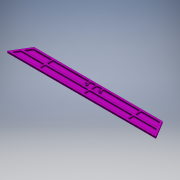
# Autodesk Inventor part: アーム　ハシゴ
Saved by Autodesk Inventor 2016 (Build 200138000, 138)
## iProperties
Created: 2016-03-06
Part Number: アーム　ハシゴ
Material: GFRP
Document SubType Name: Modeling
Designer: Takumi
Density: 1.75 g/cm^3
Appearance: 滑らか - 紫
Mass: 17.764 g
Surface Area: 193.734 cm^2
Volume: 10.1509 cm^3
Author: Takumi
Autodesk Inventor part; units mm, degrees
ref_plane "YZ Plane" through (0, 0, 0) normal (1, 0, 0) x (0, 1, 0)
ref_plane "XZ Plane" through (0, 0, 0) normal (0, 1, 0) x (-1, 0, 0)
ref_plane "XY Plane" through (0, 0, 0) normal (0, 0, 1) x (1, 0, 0)
sketch "スケッチ1" plane through (0, 0, 0) normal (0, 0, 1) x (1, 0, 0)
  line L0 (0, 0) -> (0, -14.5)
  line L1 (29.2409, -29) -> (295.7591, -29)
  line L2 (325, -16) -> (325, 0)
  line L3 (277.6805, 0.8) -> (47.3195, 0.8)
  line L4 (0, -14.5) -> (325, -14.5) construction
  arc A0 (325, -16) -> (325, -13) centre (325, -14.5) ccw
  line L5 (162.5, 0.8) -> (162.5, -29) construction
  arc A1 (161.5, -29) -> (162.5, -30) centre (162.5, -29) ccw
  line L6 (83.25, 0.8) -> (83.25, -29) construction
  arc A2 (82.25, -29) -> (83.25, -30) centre (83.25, -29) ccw
  line L7 (241.75, 0.8) -> (241.75, -29) construction
  arc A3 (240.75, -29) -> (241.75, -30) centre (241.75, -29) ccw
  line L8 (3, -3) -> (3, -13)
  line L9 (34.5698, -26) -> (82.25, -26)
  line L10 (82.25, -2.2) -> (82.25, -13)
  line L11 (82.25, -16) -> (82.25, -26)
  line L12 (84.25, -26) -> (84.25, -16)
  line L13 (84.25, -13) -> (84.25, -2.2)
  line L14 (161.5, -2.2) -> (161.5, -13)
  line L15 (161.5, -16) -> (161.5, -26)
  line L16 (163.5, -26) -> (163.5, -16)
  line L17 (163.5, -13) -> (163.5, -2.2)
  line L18 (84.25, -16) -> (161.5, -16)
  line L19 (275.9916, -2.2) -> (242.75, -2.2)
  line L20 (240.75, -2.2) -> (240.75, -13)
  line L21 (240.75, -16) -> (240.75, -26)
  line L22 (163.5, -16) -> (240.75, -16)
  line L23 (242.75, -26) -> (242.75, -16)
  line L24 (242.75, -13) -> (242.75, -2.2)
  line L25 (84.25, -26) -> (240.75, -26)
  line L26 (242.75, -26) -> (290.4302, -26)
  line L27 (322, -13) -> (322, -3)
  line L28 (150.5, 0.8) -> (150.5, -13) construction
  arc A4 (149.5, -14.5) -> (151.5, -14.5) centre (150.5, -14.5) ccw
  line L29 (174.5, -14.5) -> (174.5, 0.8) construction
  arc A5 (173.5, -14.5) -> (175.5, -14.5) centre (174.5, -14.5) ccw
  line L30 (149.5, -2.2) -> (149.5, -5.9046)
  line L31 (149.5, -11.5614) -> (149.5, -13)
  line L32 (151.5, -13) -> (151.5, -11.5614)
  line L33 (151.5, -5.9046) -> (151.5, -2.2)
  arc A6 (151.5, -11.5614) -> (151.5, -5.9046) centre (150.5, -8.733) ccw
  arc A7 (149.5, -5.9046) -> (149.5, -11.5614) centre (150.5, -8.733) ccw
  line L34 (149.5, -2.2) -> (84.25, -2.2)
  arc A8 (173.5, -5.9046) -> (173.5, -11.5614) centre (174.5, -8.733) ccw
  arc A9 (175.5, -11.5614) -> (175.5, -5.9046) centre (174.5, -8.733) ccw
  line L35 (175.5, -13) -> (175.5, -11.5614)
  line L36 (175.5, -5.9046) -> (175.5, -2.2)
  line L37 (173.5, -2.2) -> (173.5, -5.9046)
  line L38 (173.5, -11.5614) -> (173.5, -13)
  line L39 (161.5, -13) -> (151.5, -13)
  line L40 (149.5, -13) -> (84.25, -13)
  line L41 (240.75, -13) -> (175.5, -13)
  line L42 (173.5, -13) -> (163.5, -13)
  line L43 (240.75, -2.2) -> (175.5, -2.2)
  line L44 (173.5, -2.2) -> (163.5, -2.2)
  line L45 (161.5, -2.2) -> (151.5, -2.2)
  line L46 (234, 121) -> (91, 121)
  line L47 (18.0787, 0.8) -> (0, -29)
  line L48 (306.9213, 0.8) -> (325, -29)
  line L49 (162.5, 0.8) -> (162.5, 121)
  line L50 (92.6889, 118) -> (232.3111, 118)
  line L51 (40.6364, -16) -> (82.25, -16)
  line L52 (82.25, -13) -> (42.4564, -13)
  line L53 (82.25, -2.2) -> (49.0084, -2.2)
  line L54 (82.25, 100.793) -> (92.6889, 118)
  line L55 (5.3289, -26) -> (11.3956, -16)
  line L56 (13.2156, -13) -> (19.7676, -2.2)
  line L57 (282.5436, -13) -> (242.75, -13)
  line L58 (305.2324, -2.2) -> (311.7844, -13)
  line L59 (313.6044, -16) -> (319.6711, -26)
  line L60 (242.75, -16) -> (284.3636, -16)
  line L61 (342.763, -39) -> (312.551, 10.8)
  line L62 (12.449, 10.8) -> (-17.763, -39)
  line L63 (47.3195, 0.8) -> (29.2409, -29)
  line L64 (295.7591, -29) -> (277.6805, 0.8)
  line L65 (49.0084, -2.2) -> (42.4564, -13)
  line L66 (40.6364, -16) -> (34.5698, -26)
  line L67 (290.4302, -26) -> (284.3636, -16)
  line L68 (282.5436, -13) -> (275.9916, -2.2)
  point P0 (162.5, -14.5)
  point P1 (162.5, -14.1)
  point P2 (83.25, -14.1)
  point P3 (241.75, -14.1)
  point P4 (3, -24.0549)
  point P5 (322, -24.0549)
  point P6 (150.5, -7.25)
  point P7 (174.5, -6.85)
  dimension "d0" = 29
  dimension "d1" = 325
  dimension "d3" = 3
  dimension "d4" = 2
  dimension "d5" = 2
  dimension "d6" = 2
  dimension "d32" = 3
  dimension "d33" = 3
  dimension "d35" = 3
  dimension "d36" = 3
  dimension "d37" = 2
  dimension "d43" = 143
  dimension "d44" = 150
  dimension "d48" = 3
  dimension "d49" = 3
  dimension "d50" = 3
  dimension "d51" = 3
  dimension "d52" = 3
  dimension "d53" = 10
  dimension "d54" = 35
  dimension "d55" = 35
  constraints: 149 end point, 50 parallel, 30 tangent, 20 point on circle, 18 perpendicular, 18 point on line, 10 centre point, 8 midpoint, 2 coincident, 2 horizontal, 2 vertical, 1 other
  measures "d0" distance of L0.start L47.end
  measures "d1" distance of L47.end L48.end
  measures "d3" diameter of A0
  measures "d4" diameter of A1
  measures "d5" diameter of A2
  measures "d6" diameter of A3
  measures "d32" distance between parallel lines of L1 L9
  measures "d33" distance between parallel lines of L1 L25
  measures "d35" distance between parallel lines of L3 L19
  measures "d36" distance between parallel lines of L1 L26
  measures "d37" diameter of A4
  measures "d43" distance of L46.start L46.end
  measures "d44" distance between parallel lines of L1 L46
  measures "d48" distance between parallel lines of L53 L3
  measures "d49" distance between parallel lines of L3 L34
  measures "d50" distance between parallel lines of L3 L45
  measures "d51" distance between parallel lines of L3 L44
  measures "d52" distance between parallel lines of L3 L43
  measures "d53" distance between parallel lines of L47 L62
  measures "d54" distance between parallel lines of L62 L63
  measures "d55" distance between parallel lines of L61 L64
extrude "押し出し1" add sketch "スケッチ1" along normal blind 3 contours L63 L3 L64 L1 | L14 L39 L32 A6 L33 L45 | L20 L41 L35 A9 L36 L43
extrude "押し出し2" add sketch "スケッチ1" along normal blind 0.5 contours L66 L51 L11 L9 | L10 L52 L65 L53 | L12 L18 L15 L25 | L13 L34 L30 A7 L31 L40 | L16 L22 L21 L25 | L17 L44 L37 A8 L38 L42 | L68 L57 L24 L19 | L23 L60 L67 L26
extrude "押し出し3" add sketch "スケッチ1" along normal blind 3 contours L14 L39 L32 A6 L33 L45 | L17 L44 L37 A8 L38 L42
hole "穴1" at (174.5, -8.733, 0) at (150.5, -8.733, 0) direction (0, 0, 1) diameter 3 end through all
fillet "フィレット1" radius 1 18 edges at (82.25, -16, 1.75) (82.25, -2.2, 1.75) (161.5, -16, 1.75) (161.5, -26, 1.75) (82.25, -26, 1.75) (82.25, -13, 1.75) (84.25, -13, 1.75) (84.25, -16, 1.75) (84.25, -2.2, 1.75) (84.25, -26, 1.75) (163.5, -16, 1.75) (163.5, -26, 1.75) (240.75, -26, 1.75) (240.75, -16, 1.75) (242.75, -26, 1.75) (242.75, -16, 1.75) (242.75, -13, 1.75) (242.75, -2.2, 1.75)
extrude "押し出し4" cut sketch "スケッチ1" along normal blind 3 contours L14 L39 L32 A6 L33 L45 | L17 L44 L37 A8 L38 L42 | L20 L41 L35 A9 L36 L43
extrude "押し出し5" add sketch "スケッチ1" along normal blind 0.5 contours L14 L39 L32 A6 L33 L45 | L17 L44 L37 A8 L38 L42 | L20 L41 L35 A9 L36 L43
fillet "フィレット3" radius 1 22 edges at (173.5, -2.2, 1.75) (173.5, -5.9046, 1.75) (173.5, -11.5614, 1.75) (175.5, -13, 1.75) (173.5, -13, 1.75) (175.5, -11.5614, 1.75) (175.5, -5.9046, 1.75) (175.5, -2.2, 1.75) (163.5, -2.2, 1.75) (161.5, -2.2, 1.75) (161.5, -13, 1.75) (163.5, -13, 1.75) (240.75, -13, 1.75) (240.75, -2.2, 1.75) (149.5, -11.5614, 1.75) (149.5, -13, 1.75) (151.5, -13, 1.75) (151.5, -11.5614, 1.75) (149.5, -5.9046, 1.75) (149.5, -2.2, 1.75) (151.5, -2.2, 1.75) (151.5, -5.9046, 1.75)
fillet "フィレット4" radius 1 8 edges at (49.0084, -2.2, 1.75) (40.6364, -16, 1.75) (34.5698, -26, 1.75) (42.4564, -13, 1.75) (284.3636, -16, 1.75) (275.9916, -2.2, 1.75) (282.5436, -13, 1.75) (290.4302, -26, 1.75)
equation "\"d33\" = d31"
equation "\"d8\" = 0.5 * d7"
equation "\"d10\" = 0.5 * d9"
equation "\"d34\" = d31"
equation "\"d31\" = 3"
equation "\"d7\" = 158.5"
equation "\"d9\" = 158.5"
